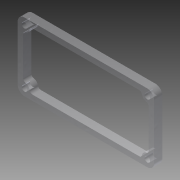
# Autodesk Inventor part: AcrylicLowerCore
Saved by Autodesk Inventor 2014 SP1 (Build 180222100, 222)
## iProperties
Created: 2016-03-18
Part Number: AcrylicLowerCore
Material: Acrylic, Clear
Document SubType Name: Modeling
Designer: Tyler
Density: 1.19 g/cm^3
Appearance: Transparent - Clear
Author: Tyler
Autodesk Inventor part; units mm, degrees
ref_plane "YZ Plane" through (0, 0, 0) normal (1, 0, 0) x (0, 1, 0)
ref_plane "XZ Plane" through (0, 0, 0) normal (0, 1, 0) x (-1, 0, 0)
ref_plane "XY Plane" through (0, 0, 0) normal (0, 0, 1) x (1, 0, 0)
sketch "Sketch1" plane through (0, 0, 0) normal (0, 1, 0) x (-1, 0, 0)
  line L0 (50, 25) -> (-50, 25)
  line L1 (-50, 25) -> (-50, -25)
  line L2 (-50, -25) -> (50, -25)
  line L3 (50, -25) -> (50, 25)
  line L4 (50, 25) -> (-50, -25) construction
  line L5 (-50, 25) -> (50, -25) construction
  point P0 (0, 0)
  dimension "d0" = 100
  dimension "d1" = 50
  constraints: 12 end point, 2 midpoint, 2 parallel, 1 horizontal, 1 perpendicular
  measures "d0" distance of L2.end L1.end
  measures "d1" distance of L1.end L0.end
extrude "Extrusion1" add sketch "Sketch1" along normal blind 6
fillet "Fillet1" radius 5 4 edges at (50, 3, 25) (50, 3, -25) (-50, 3, -25) (-50, 3, 25)
sketch "Sketch2" plane through (0, 6, 0) normal (0, 1, 0) x (1, 0, 0)
  line L0 (-39.5, -21.25) -> (-30.5, -21.25)
  line L1 (-30.5, -21.25) -> (-30.5, -4.75)
  line L2 (-30.5, -4.75) -> (-39.5, -4.75)
  line L3 (-39.5, -4.75) -> (-39.5, -21.25)
  line L4 (-39.5, -21.25) -> (-30.5, -4.75) construction
  line L5 (-30.5, -21.25) -> (-39.5, -4.75) construction
  line L6 (-25.5, -21.25) -> (-16.5, -21.25)
  line L7 (-16.5, -21.25) -> (-16.5, -4.75)
  line L8 (-16.5, -4.75) -> (-25.5, -4.75)
  line L9 (-25.5, -4.75) -> (-25.5, -21.25)
  line L10 (-25.5, -21.25) -> (-16.5, -4.75) construction
  line L11 (-16.5, -21.25) -> (-25.5, -4.75) construction
  line L12 (-11.5, -21.25) -> (-2.5, -21.25)
  line L13 (-2.5, -21.25) -> (-2.5, -4.75)
  line L14 (-2.5, -4.75) -> (-11.5, -4.75)
  line L15 (-11.5, -4.75) -> (-11.5, -21.25)
  line L16 (-11.5, -21.25) -> (-2.5, -4.75) construction
  line L17 (-2.5, -21.25) -> (-11.5, -4.75) construction
  line L18 (2.5, -21.25) -> (11.5, -21.25)
  line L19 (11.5, -21.25) -> (11.5, -4.75)
  line L20 (11.5, -4.75) -> (2.5, -4.75)
  line L21 (2.5, -4.75) -> (2.5, -21.25)
  line L22 (2.5, -21.25) -> (11.5, -4.75) construction
  line L23 (11.5, -21.25) -> (2.5, -4.75) construction
  line L24 (16.5, -21.25) -> (25.5, -21.25)
  line L25 (25.5, -21.25) -> (25.5, -4.75)
  line L26 (25.5, -4.75) -> (16.5, -4.75)
  line L27 (16.5, -4.75) -> (16.5, -21.25)
  line L28 (16.5, -21.25) -> (25.5, -4.75) construction
  line L29 (25.5, -21.25) -> (16.5, -4.75) construction
  line L30 (30.5, -21.25) -> (39.5, -21.25)
  line L31 (39.5, -21.25) -> (39.5, -4.75)
  line L32 (39.5, -4.75) -> (30.5, -4.75)
  line L33 (30.5, -4.75) -> (30.5, -21.25)
  line L34 (30.5, -21.25) -> (39.5, -4.75) construction
  line L35 (39.5, -21.25) -> (30.5, -4.75) construction
  point P0 (0, 0)
  point P1 (-35, -13)
  point P2 (-21, -13)
  point P3 (-7, -13)
  point P4 (7, -13)
  point P5 (21, -13)
  point P6 (35, -13)
  dimension "d5" = 9
  dimension "d6" = 16.5
  dimension "d9" = 14
  dimension "d14" = 7
  dimension "d15" = 13
  constraints: 72 end point, 12 midpoint, 2 horizontal, 2 parallel, 1 collinear, 1 perpendicular, 54 other
  measures "d5" distance of L1.end L2.end
  measures "d6" distance of L0.end L1.end
  measures "d9" distance of L0.end L7.start
  measures "d14" horizontal distance of point (7, -13) point (0, 0)
  measures "d15" vertical distance of point (7, -13) point (0, 0)
extrude "Extrusion2" [suppressed]
sketch "Sketch3" plane through (0, 6, 0) normal (0, 1, 0) x (1, 0, 0)
  line L0 (-16.5, -21.25) -> (-25.5, -21.25) projected
  line L1 (-45, -25) -> (45, -25) projected
  line L2 (45, 25) -> (-45, 25) projected
  line L3 (-38, 1) -> (-32, 1)
  line L4 (-32, 1) -> (-32, 21)
  line L5 (-32, 21) -> (-38, 21)
  line L6 (-38, 21) -> (-38, 1)
  line L7 (-38, 1) -> (-32, 21) construction
  line L8 (-32, 1) -> (-38, 21) construction
  line L9 (-24, 1) -> (-18, 1)
  line L10 (-18, 1) -> (-18, 21)
  line L11 (-18, 21) -> (-24, 21)
  line L12 (-24, 21) -> (-24, 1)
  line L13 (-24, 1) -> (-18, 21) construction
  line L14 (-18, 1) -> (-24, 21) construction
  line L15 (-10, 1) -> (-4, 1)
  line L16 (-4, 1) -> (-4, 21)
  line L17 (-4, 21) -> (-10, 21)
  line L18 (-10, 21) -> (-10, 1)
  line L19 (-10, 1) -> (-4, 21) construction
  line L20 (-4, 1) -> (-10, 21) construction
  line L21 (4, 1) -> (10, 1)
  line L22 (10, 1) -> (10, 21)
  line L23 (10, 21) -> (4, 21)
  line L24 (4, 21) -> (4, 1)
  line L25 (4, 1) -> (10, 21) construction
  line L26 (10, 1) -> (4, 21) construction
  line L27 (18, 1) -> (24, 1)
  line L28 (24, 1) -> (24, 21)
  line L29 (24, 21) -> (18, 21)
  line L30 (18, 21) -> (18, 1)
  line L31 (18, 1) -> (24, 21) construction
  line L32 (24, 1) -> (18, 21) construction
  line L33 (32, 1) -> (38, 1)
  line L34 (38, 1) -> (38, 21)
  line L35 (38, 21) -> (32, 21)
  line L36 (32, 21) -> (32, 1)
  line L37 (32, 1) -> (38, 21) construction
  line L38 (38, 1) -> (32, 21) construction
  point P0 (0, 0)
  point P1 (-35, 11)
  point P2 (-21, 11)
  point P3 (-7, 11)
  point P4 (7, 11)
  point P5 (21, 11)
  point P6 (35, 11)
  dimension "d20" = 14
  dimension "d25" = 7
  dimension "d26" = 6
  dimension "d27" = 20
  dimension "d28" = 4
  dimension "d29" = 3.75
  constraints: 72 end point, 12 midpoint, 2 horizontal, 2 parallel, 1 collinear, 1 perpendicular, 54 other
  measures "d20" distance of L3.start L9.start
  measures "d25" horizontal distance of point (-7, 11) point (0, 0)
  measures "d26" distance of L4.end L5.end
  measures "d27" distance between parallel lines of L5 L3
  measures "d28" distance between parallel lines of L11 L2
  measures "d29" distance between parallel lines of L1 L0
extrude "Extrusion3" [suppressed]
sketch "Sketch4" plane through (0, 6, 0) normal (0, 1, 0) x (1, 0, 0)
  arc A0 (-50, -20) -> (-45, -25) centre (-45, -20) ccw projected
  arc A1 (45, -25) -> (50, -20) centre (45, -20) ccw projected
  arc A2 (50, 20) -> (45, 25) centre (45, 20) ccw projected
  arc A3 (-45, 25) -> (-50, 20) centre (-45, 20) ccw projected
  point P0 (0, 0)
  constraints: 4 coincident
hole "Hole1" at (-45, 6, -20) at (45, 6, -20) at (45, 6, 20) at (-45, 6, 20) direction (0, -1, 0) diameter 4 end through all
sketch "Sketch5" plane through (0, 6, 0) normal (0, 1, 0) x (1, 0, 0)
  circle A0 centre (45, -20) radius 2 projected
  circle A1 centre (-45, 20) radius 2 projected
  circle A2 centre (45, 20) radius 2 projected
  circle A3 centre (-45, -20) radius 2 projected
  line L0 (24, 21) -> (24, 1) projected
  line L1 (24, 1) -> (18, 1) projected
  line L2 (18, 1) -> (18, 21) projected
  line L3 (18, 21) -> (24, 21) projected
  line L4 (-4, 21) -> (-4, 1) projected
  line L5 (-4, 1) -> (-10, 1) projected
  line L6 (-10, 1) -> (-10, 21) projected
  line L7 (-10, 21) -> (-4, 21) projected
  line L8 (-32, 21) -> (-32, 1) projected
  line L9 (-32, 1) -> (-38, 1) projected
  line L10 (-38, 1) -> (-38, 21) projected
  line L11 (-38, 21) -> (-32, 21) projected
  line L12 (-18, 21) -> (-18, 1) projected
  line L13 (-18, 1) -> (-24, 1) projected
  line L14 (-24, 1) -> (-24, 21) projected
  line L15 (-24, 21) -> (-18, 21) projected
  line L16 (10, 21) -> (10, 1) projected
  line L17 (10, 1) -> (4, 1) projected
  line L18 (4, 1) -> (4, 21) projected
  line L19 (4, 21) -> (10, 21) projected
  line L20 (38, 21) -> (38, 1) projected
  line L21 (38, 1) -> (32, 1) projected
  line L22 (32, 1) -> (32, 21) projected
  line L23 (32, 21) -> (38, 21) projected
  line L24 (-45, -25) -> (45, -25) projected
  line L25 (50, -20) -> (50, 20) projected
  line L26 (45, 25) -> (-45, 25) projected
  line L27 (-50, 20) -> (-50, -20) projected
  line L28 (-39.0839, 21) -> (39.0839, 21)
  line L29 (-46, -14.0839) -> (-46, 14.0839)
  arc A4 (-44.3333, 16.0559) -> (-41.0559, 19.3333) centre (-45, 20) ccw
  arc A5 (41.0559, 19.3333) -> (44.3333, 16.0559) centre (45, 20) ccw
  arc A6 (44.3333, -16.0559) -> (41.0559, -19.3333) centre (45, -20) ccw
  arc A7 (-41.0559, -19.3333) -> (-44.3333, -16.0559) centre (-45, -20) ccw
  line L30 (46, 14.0839) -> (46, -14.0839)
  line L31 (39.0839, -21) -> (-39.0839, -21)
  arc A8 (41.0559, 19.3333) -> (39.0839, 21) centre (39.0839, 19) ccw
  arc A9 (46, 14.0839) -> (44.3333, 16.0559) centre (44, 14.0839) ccw
  arc A10 (44.3333, -16.0559) -> (46, -14.0839) centre (44, -14.0839) ccw
  arc A11 (39.0839, -21) -> (41.0559, -19.3333) centre (39.0839, -19) ccw
  arc A12 (-41.0559, -19.3333) -> (-39.0839, -21) centre (-39.0839, -19) ccw
  arc A13 (-46, -14.0839) -> (-44.3333, -16.0559) centre (-44, -14.0839) ccw
  arc A14 (-39.0839, 21) -> (-41.0559, 19.3333) centre (-39.0839, 19) ccw
  arc A15 (-44.3333, 16.0559) -> (-46, 14.0839) centre (-44, 14.0839) ccw
  point P0 (0, 0)
  point P1 (41.127, 21)
  point P2 (41.127, -21)
  point P3 (-46, -16.127)
  point P4 (-46, 16.127)
  point P5 (46, 16.127)
  point P6 (46, -16.127)
  point P7 (-41.127, -21)
  point P8 (-41.127, 21)
  dimension "d39" = 4
  dimension "d40" = 8
  dimension "d41" = 8
  dimension "d42" = 8
  dimension "d43" = 8
  dimension "d44" = 4
  dimension "d45" = 4
  dimension "d46" = 4
  dimension "d47" = 2
  constraints: 32 point on circle, 16 tangent, 12 centre point, 8 end point, 8 point on line, 7 equal radius
  measures "d39" distance between parallel lines of L28 L26
  measures "d40" diameter of A4
  measures "d41" diameter of A7
  measures "d42" diameter of A6
  measures "d43" diameter of A5
  measures "d44" distance between parallel lines of L27 L29
  measures "d45" distance between parallel lines of L24 L31
  measures "d46" distance between parallel lines of L25 L30
  measures "d47" radius of A8
extrude "Extrusion4" cut sketch "Sketch5" against normal blind 10 contours L28 L22 L21 L20 A8 A5 A9 L30 A10 A6 A11 L31 A12 A7 A13 L29 A15 A4 A14 L10 L9 L8 L14 L13 L12 L6 L5 L4 L18 L17 L16 L2 L1 L0 | L0 L1 L2 L3 | L23 L20 L21 L22 | L16 L17 L18 L19 | L4 L5 L6 L7 | L12 L13 L14 L15 | L8 L9 L10 L11
equation "\"d14\" = 0.5 * d9"
equation "\"d25\" = 0.5 * d20"
body "Solid1"
